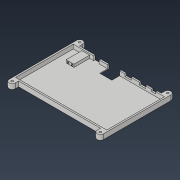
# Autodesk Inventor part: Display 5inch Housing
Saved by Autodesk Inventor 2022.3 (Build 263350000, 350)
## iProperties
Part Number: Display 5inch Housing
Material: Generisch
Document SubType Name: Modeling
Designer: rYan
Density: 1 g/cm^3
Appearance: Vorgabe
Author: rYan
Autodesk Inventor part; units mm, degrees
ref_plane "YZ Plane" through (0, 0, 0) normal (1, 0, 0) x (0, 1, 0)
ref_plane "XZ Plane" through (0, 0, 0) normal (0, 1, 0) x (-1, 0, 0)
ref_plane "XY Plane" through (0, 0, 0) normal (0, 0, 1) x (1, 0, 0)
sketch "Skizze1" plane through (0, 0, 0) normal (0, 0, 1) x (1, 0, 0)
  line L0 (-52.5, 39) -> (52.5, 39)
  line L1 (-52.5, -39) -> (52.5, -39)
  line L2 (52.5, -39) -> (52.5, -43.25)
  line L3 (-52.5, -39) -> (-52.5, -43.25)
  line L4 (-60.5, -43.25) -> (-60.5, 43.25)
  line L5 (-52.5, 39) -> (-52.5, 43.25)
  line L6 (52.5, 39) -> (52.5, 43.25)
  line L7 (60.5, 43.25) -> (60.5, -43.25)
  arc A0 (-52.5, 43.25) -> (-60.5, 43.25) centre (-56.5, 43.25) ccw
  arc A1 (60.5, 43.25) -> (52.5, 43.25) centre (56.5, 43.25) ccw
  arc A2 (52.5, -43.25) -> (60.5, -43.25) centre (56.5, -43.25) ccw
  arc A3 (-60.5, -43.25) -> (-52.5, -43.25) centre (-56.5, -43.25) ccw
  line L8 (0, 66.15) -> (0, -66.15) construction
  line L9 (-84.7, 0) -> (84.7, 0) construction
  circle A4 centre (-56.5, 43.25) radius 1.4
  circle A5 centre (56.5, 43.25) radius 1.4
  circle A6 centre (56.5, -43.25) radius 1.4
  circle A7 centre (-56.5, -43.25) radius 1.4
  point P0 (0, 0)
  dimension "d0" = 121
  dimension "d1" = 78
  dimension "d2" = 8
  dimension "d3" = 86.5
  dimension "d4" = 2.8
  constraints: 16 end point, 8 centre point, 8 point on circle, 8 tangent, 5 vertical, 4 coincident, 2 horizontal, 1 collinear, 1 perpendicular, 10 other
  measures "d0" distance between parallel lines of L7 L4
  measures "d1" distance between parallel lines of L1 L0
  measures "d2" distance between parallel lines of L7 L6
  measures "d3" distance of A2.centre A1.centre
  measures "d4" diameter of A4
extrude "Extrusion1" add sketch "Skizze1" along normal blind 1.1
sketch "Skizze8" plane through (0, 0, 1.1) normal (0, 0, 1) x (1, 0, 0)
  line L0 (-58.5, -37) -> (58.5, -37)
  line L1 (58.5, -37) -> (58.5, 37)
  line L2 (58.5, 37) -> (-58.5, 37)
  line L3 (-58.5, 37) -> (-58.5, -37)
  line L4 (-58.5, -37) -> (58.5, 37) construction
  line L5 (58.5, -37) -> (-58.5, 37) construction
  line L6 (60.5, -43.25) -> (60.5, 43.25) projected
  line L7 (52.5, 39) -> (-52.5, 39) projected
  line L8 (-60.5, 43.25) -> (-60.5, -43.25) projected
  arc A0 (-60.5, -43.25) -> (-52.5, -43.25) centre (-56.5, -43.25) ccw projected
  line L9 (-52.5, -43.25) -> (-52.5, -39) projected
  line L10 (-52.5, -39) -> (52.5, -39) projected
  line L11 (52.5, -39) -> (52.5, -43.25) projected
  arc A1 (52.5, -43.25) -> (60.5, -43.25) centre (56.5, -43.25) ccw projected
  line L12 (60.5, -43.25) -> (60.5, 43.25) projected
  arc A2 (60.5, 43.25) -> (52.5, 43.25) centre (56.5, 43.25) ccw projected
  line L13 (52.5, 43.25) -> (52.5, 39) projected
  line L14 (52.5, 39) -> (-52.5, 39) projected
  line L15 (-52.5, 39) -> (-52.5, 43.25) projected
  arc A3 (-52.5, 43.25) -> (-60.5, 43.25) centre (-56.5, 43.25) ccw projected
  circle A4 centre (-56.5, -43.25) radius 1.4 projected
  circle A5 centre (56.5, -43.25) radius 1.4 projected
  circle A6 centre (56.5, 43.25) radius 1.4 projected
  circle A7 centre (-56.5, 43.25) radius 1.4 projected
  point P0 (0, 0)
  dimension "d45" = 2
  dimension "d46" = 2
  constraints: 12 end point, 2 midpoint, 2 parallel, 1 horizontal, 1 perpendicular
  measures "d45" distance between parallel lines of L6 L1
  measures "d46" distance between parallel lines of L7 L2
extrude "Extrusion8" add sketch "Skizze8" along normal blind 5.4
sketch "Skizze9" plane through (-52.5, 39, 0) normal (0, 1, 0) x (1, 0, 0)
  line L0 (105, -6.5) -> (0, -6.5) projected
  line L1 (-6, -6.5) -> (111, -6.5) projected
  line L2 (99.9, -6.5) -> (94.5, -6.5)
  line L3 (94.5, -6.5) -> (94.5, -4.1)
  line L4 (94.5, -4.1) -> (99.9, -4.1)
  line L5 (99.9, -4.1) -> (99.9, -6.5)
  line L6 (86.95, -6.5) -> (78.95, -6.5)
  line L7 (78.95, -6.5) -> (78.95, -3.5)
  line L8 (78.95, -3.5) -> (86.95, -3.5)
  line L9 (86.95, -3.5) -> (86.95, -6.5)
  line L10 (68.25, -6.5) -> (60.25, -6.5)
  line L11 (60.25, -6.5) -> (60.25, -3.5)
  line L12 (60.25, -3.5) -> (68.25, -3.5)
  line L13 (68.25, -3.5) -> (68.25, -6.5)
  line L14 (53.5, -6.5) -> (37.9, -6.5)
  line L15 (37.9, -6.5) -> (37.9, 0.5)
  line L16 (37.9, 0.5) -> (53.5, 0.5)
  line L17 (53.5, 0.5) -> (53.5, -6.5)
  line L18 (20.2, -6.5) -> (27.2, -6.5)
  line L19 (27.2, -6.5) -> (27.2, -1.1)
  line L20 (27.2, -1.1) -> (20.2, -1.1)
  line L21 (20.2, -1.1) -> (20.2, -6.5)
  line L22 (97.2, -4.1) -> (97.2, -6.5) construction
  line L23 (82.95, -3.5) -> (82.95, -6.5) construction
  line L24 (64.25, -3.5) -> (64.25, -6.5) construction
  line L25 (45.7, 0.5) -> (45.7, -6.5) construction
  line L26 (23.7, -1.1) -> (23.7, -6.5) construction
  line L27 (105, 0) -> (105, -6.5) construction
  line L28 (37.9, -6.5) -> (27.2, -6.5)
  line L29 (27.2, -6.5) -> (27.2, -5.5)
  line L30 (27.2, -5.5) -> (37.9, -5.5)
  line L31 (37.9, -5.5) -> (37.9, -6.5)
  point P0 (52.5, 0)
  point P1 (27.2, -6.5)
  point P2 (94.5, -6.5)
  point P3 (99.9, -6.5)
  dimension "d49" = 7.8
  dimension "d50" = 22.05
  dimension "d51" = 40.75
  dimension "d52" = 59.3
  dimension "d53" = 81.3
  dimension "d54" = 2.4
  dimension "d55" = 3
  dimension "d56" = 7
  dimension "d57" = 5.4
  dimension "d58" = 5.4
  dimension "d59" = 8
  dimension "d60" = 8
  dimension "d61" = 15.6
  dimension "d62" = 7
  dimension "d65" = 1
  constraints: 58 end point, 12 parallel, 10 midpoint, 7 point on line, 6 horizontal, 6 perpendicular
  measures "d49" distance between parallel lines of L22 L27
  measures "d50" distance between parallel lines of L23 L27
  measures "d51" distance between parallel lines of L24 L27
  measures "d52" distance between parallel lines of L25 L27
  measures "d53" distance between parallel lines of L26 L27
  measures "d54" distance of L2.end L3.end
  measures "d55" distance of L6.end L7.end
  measures "d56" distance of L14.end L15.end
  measures "d57" distance of L20.end L18.start
  measures "d58" distance of L3.end L4.end
  measures "d59" distance of L7.end L8.end
  measures "d60" distance of L11.end L12.end
  measures "d61" distance of L15.end L16.end
  measures "d62" distance of L19.end L20.end
  measures "d65" distance between parallel lines of L0 L30
extrude "Extrusion9" cut sketch "Skizze9" against normal blind 12
sketch "Skizze11" plane through (0, 0, 1.1) normal (0, 0, 1) x (1, 0, 0)
  line L0 (-58.5, 37) -> (-32.3, 37) projected
  line L1 (-37.5, 37) -> (-47.5, 37)
  line L2 (-47.5, 37) -> (-47.5, 17)
  line L3 (-47.5, 17) -> (-37.5, 17)
  line L4 (-37.5, 17) -> (-37.5, 37)
  line L5 (-52.5, 39) -> (-52.5, 43.25) projected
  point P0 (0, 0)
  point P1 (-42.5, 37)
  dimension "d66" = 10
  dimension "d67" = 10
  dimension "d68" = 20
  constraints: 8 end point, 2 parallel, 1 horizontal, 1 midpoint, 1 perpendicular, 1 point on line
  measures "d66" distance of L2.end L3.end
  measures "d67" distance from line of point (-42.5, 37) L5
  measures "d68" distance of L1.end L2.end
extrude "Extrusion10" add sketch "Skizze11" along normal blind 3.6
sketch "Skizze12" plane through (-52.5, 39, 6.5) normal (0, 1, 0) x (1, 0, 0)
  line L0 (5, 5.4) -> (5, 1.8) projected
  line L1 (15, 5.4) -> (5, 5.4) projected
  line L2 (15, 5.4) -> (15, 1.8) projected
  line L3 (10, 5.4) -> (10, 0) construction
  line L4 (13.6, 5) -> (11.4, 5)
  line L5 (11.4, 5) -> (11.4, 2.8)
  line L6 (11.4, 2.8) -> (13.6, 2.8)
  line L7 (13.6, 2.8) -> (13.6, 5)
  line L8 (13.6, 5) -> (11.4, 2.8) construction
  line L9 (11.4, 5) -> (13.6, 2.8) construction
  line L10 (8.6, 5) -> (6.4, 5)
  line L11 (6.4, 5) -> (6.4, 2.8)
  line L12 (6.4, 2.8) -> (8.6, 2.8)
  line L13 (8.6, 2.8) -> (8.6, 5)
  line L14 (8.6, 5) -> (6.4, 2.8) construction
  line L15 (6.4, 5) -> (8.6, 2.8) construction
  line L16 (5, 1.8) -> (15, 1.8) projected
  point P0 (52.5, 6.5)
  point P1 (12.5, 3.9)
  point P2 (7.5, 3.9)
  point P3 (7.5, 3.9)
  point P4 (12.5, 3.9)
  point P5 (8.6, 5.4)
  point P6 (6.4, 5.4)
  point P7 (13.6, 5.4)
  point P8 (11.4, 5.4)
  point P9 (7.5, 3.9)
  dimension "d73" = 5
  dimension "d74" = 2.2
  dimension "d75" = 2.2
  dimension "d78" = 1.5
  constraints: 26 end point, 8 midpoint, 4 parallel, 2 horizontal, 2 perpendicular, 1 symmetric about line, 2 other
  measures "d73" distance of point (7.5, 3.9) point (12.5, 3.9)
  measures "d74" distance of L10.end L11.end
  measures "d75" distance of L11.end L12.end
  measures "d78" distance from line of L1 point (7.5, 3.9)
extrude "Extrusion11" cut sketch "Skizze12" against normal up to surface (22 mm away) contours L7 L6 L5 L4 | L13 L12 L11 L10
sketch "Skizze13" plane through (-52.5, 39, 6.5) normal (0, 1, 0) x (1, 0, 0)
  line L0 (13.6, 2.8) -> (11.4, 2.8) construction
  line L1 (11.4, 5) -> (13.6, 5) construction
  line L2 (8.6, 2.8) -> (6.4, 2.8) construction
  line L3 (6.4, 5) -> (8.6, 5) construction
  line L4 (7.5, 2.8) -> (7.5, 5) construction
  line L5 (8.6, 5) -> (6.4, 5) construction
  line L6 (12.5, 5) -> (12.5, 2.8) construction
  line L7 (14, 5.4) -> (11, 5.4)
  line L8 (11, 5.4) -> (11, 2.4)
  line L9 (11, 2.4) -> (14, 2.4)
  line L10 (14, 2.4) -> (14, 5.4)
  line L11 (14, 5.4) -> (11, 2.4) construction
  line L12 (11, 5.4) -> (14, 2.4) construction
  line L13 (9, 5.4) -> (6, 5.4)
  line L14 (6, 5.4) -> (6, 2.4)
  line L15 (6, 2.4) -> (9, 2.4)
  line L16 (9, 2.4) -> (9, 5.4)
  line L17 (9, 5.4) -> (6, 2.4) construction
  line L18 (6, 5.4) -> (9, 2.4) construction
  point P0 (52.5, 6.5)
  point P1 (12.5, 3.9)
  point P2 (7.5, 3.9)
  dimension "d79" = 3
  dimension "d80" = 3
  dimension "d81" = 3
  dimension "d82" = 3
  constraints: 28 end point, 10 midpoint, 4 parallel, 2 horizontal, 2 perpendicular
  measures "d79" distance of L9.end L8.end
  measures "d80" distance of L8.end L7.end
  measures "d81" distance of L15.end L14.end
  measures "d82" distance of L14.end L13.end
extrude "Extrusion12" cut sketch "Skizze13" against normal blind 10
equation "\"d60\" = d59"
